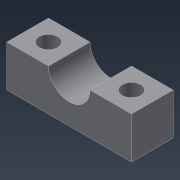
# Autodesk Inventor part: P014-Chapeau_bielle
Saved by Autodesk Inventor 2021.3 (Build 253353000, 353)
## iProperties
Created: 2022-03-31
Part Number: P014-Chapeau_bielle
Material: Générique
Document SubType Name: Modeling
Designer: remi
Density: 1 g/cm^3
Appearance: Par défaut
Author: remi
Autodesk Inventor part; units mm, degrees
ref_plane "YZ Plane" through (0, 0, 0) normal (1, 0, 0) x (0, 1, 0)
ref_plane "XZ Plane" through (0, 0, 0) normal (0, 1, 0) x (-1, 0, 0)
ref_plane "XY Plane" through (0, 0, 0) normal (0, 0, 1) x (1, 0, 0)
sketch "Sketch2" plane through (0, 0, 0) normal (0, 1, 0) x (-1, 0, 0)
  line L0 (5, 0) -> (15, 0)
  line L1 (15, 0) -> (15, -10)
  line L2 (15, -10) -> (-15, -10)
  line L3 (-15, -10) -> (-15, 0)
  line L4 (-15, 0) -> (-5, 0)
  arc A0 (-5, 0) -> (5, 0) centre (0, 0) ccw
  dimension "d0" = 10
  dimension "d1" = 5
  dimension "d12" = 10
  constraints: 10 end point, 3 perpendicular, 2 point on circle, 2 point on line, 1 centre point, 1 coincident, 1 collinear, 1 horizontal, 1 horizontal alignment
  measures "d0" distance of L0.start L0.end
  measures "d1" radius of A0
  measures "d12" distance from line of A0.centre L2
extrude "Extrusion1" add sketch "Sketch2" along normal blind 10
sketch "Sketch3" plane through (0, 0, 0) normal (0, 0, 1) x (1, 0, 0)
  line L0 (5, 0) -> (15, 0) construction
  line L1 (15, 0) -> (15, 10) construction
  line L2 (5, 10) -> (15, 10) construction
  line L3 (5, 0) -> (5, 10) construction
  line L4 (-15, 0) -> (-5, 0) construction
  line L5 (-5, 0) -> (-5, 10) construction
  line L6 (-15, 10) -> (-5, 10) construction
  line L7 (-15, 0) -> (-15, 10) construction
  line L8 (15, 10) -> (5, 0) construction
  line L9 (5, 10) -> (15, 0) construction
  line L10 (-5, 0) -> (-15, 10) construction
  line L11 (-5, 10) -> (-15, 0) construction
  point P0 (0, 0)
  point P1 (-10, 5)
  point P2 (10, 5)
  constraints: 8 end point, 2 midpoint, 2 perpendicular, 1 parallel
hole "Hole1" at (-10, 5, 0) at (10, 5, 0) direction (0, 0, -1) diameter 4.5 end through all clearance for "Flat Head Machine Screw" size "M4" standard "Ansi Metric M Profile"
body "Solid1"
